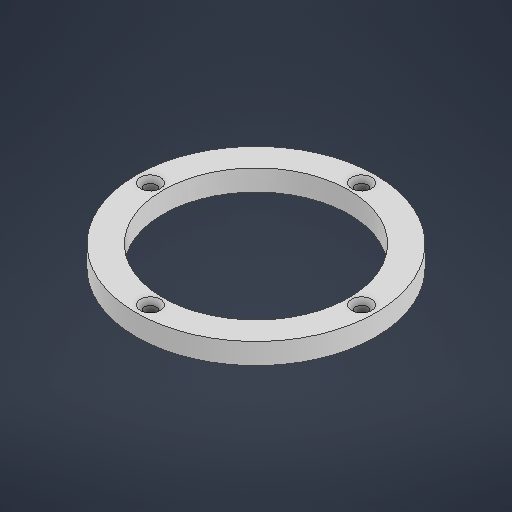
# Autodesk Inventor part: innerbearingwheel
Saved by Autodesk Inventor 2026 (Build 300175000, 175)
## iProperties
Created: 2026-04-15
Part Number: innerbearingwheel
Material: Generic
Document SubType Name: Modeling
Designer: CAD237 PC35
Density: 1 g/cm^3
Appearance: Default
Author: CAD237 PC35
Autodesk Inventor part; units mm, degrees
ref_plane "YZ Plane" through (0, 0, 0) normal (1, 0, 0) x (0, 1, 0)
ref_plane "XZ Plane" through (0, 0, 0) normal (0, 1, 0) x (-1, 0, 0)
ref_plane "XY Plane" through (0, 0, 0) normal (0, 0, 1) x (1, 0, 0)
sketch "Sketch1" plane through (0, 0, 0) normal (0, 1, 0) x (-1, 0, 0)
  circle A0 centre (0, 0) radius 57.15
  circle A1 centre (0, 0) radius 44.5
  dimension "d0" = 114.3
  dimension "d1" = 89
  constraints: 2 centre point, 2 coincident
  measures "d0" diameter of A0
  measures "d1" diameter of A1
extrude "Extrusion1" add sketch "Sketch1" along normal blind 10
sketch "Sketch3" plane through (0, 10, 0) normal (0, 1, 0) x (1, 0, 0)
  line L0 (0, 0) -> (0, -50.4952)
  point P0 (50.4952, 0)
  point P1 (50.4952, 0)
  point P2 (0, 50.4952)
  point P3 (0, 50.4952)
  point P4 (-50.4952, 0)
  point P5 (-50.4952, 0)
  dimension "d18" = 50.4952
  dimension "d21" = 360
  constraints: 4 coincident, 2 end point, 1 vertical, 9 other
  measures "d18" distance of L0.start L0.end
hole "Hole1" at (0, 10, 50.4952) at (50.4952, 10, 0) at (0, 10, -50.4952) at (-50.4952, 10, 0) direction (0, -1, 0) diameter 5.7 depth 15.6718 tip angle 118 countersink diameter 9.525 countersink angle 82
body "Solid1"
